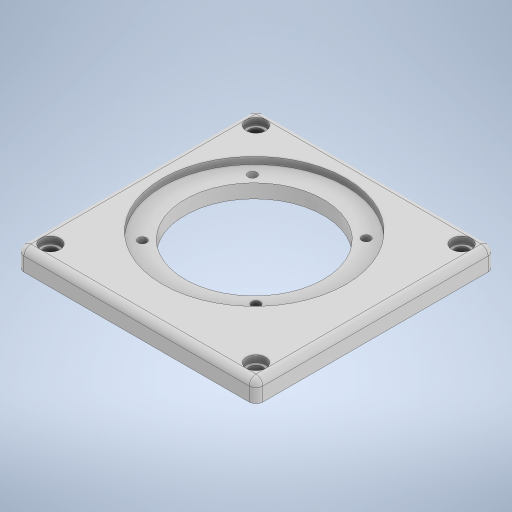
# Autodesk Inventor part: joystickBOXtop
Saved by Autodesk Inventor 2023 (Build 270158000, 158)
## iProperties
Created: 2023-09-26
Part Number: joystickBOXtop
Material: Generic
Document SubType Name: Modeling
Designer: Nikita
Density: 1 g/cm^3
Appearance: Default
Author: Nikita
Autodesk Inventor part; units mm, degrees
ref_plane "YZ Plane" through (0, 0, 0) normal (1, 0, 0) x (0, 1, 0)
ref_plane "XZ Plane" through (0, 0, 0) normal (0, 1, 0) x (-1, 0, 0)
ref_plane "XY Plane" through (0, 0, 0) normal (0, 0, 1) x (1, 0, 0)
sketch "Sketch1" plane through (0, 0, 0) normal (0, 1, 0) x (-1, 0, 0)
  line L0 (0, 0) -> (69, 0)
  line L1 (69, 0) -> (69, -69)
  line L2 (69, -69) -> (0, -69)
  line L3 (0, -69) -> (0, 0)
  dimension "d0" = 69
  dimension "d1" = 69
  constraints: 8 end point, 3 perpendicular, 1 horizontal
  measures "d0" distance of L0.start L0.end
  measures "d1" distance of L0.end L1.end
extrude "Extrusion1" add sketch "Sketch1" along normal blind 6
sketch "Sketch2" plane through (0, 6, 0) normal (0, 1, 0) x (1, 0, 0)
  line L0 (0, 0) -> (0, 69) construction
  line L1 (0, 69) -> (-69, 69) construction
  line L2 (0, 0) -> (-69, 69) construction
  line L3 (-69, 69) -> (-69, 0) construction
  line L4 (-69.6585, 0.6585) -> (-0.6585, 69.6585) construction
  circle A0 centre (-37.9036, 37.4036) radius 20
  line L5 (-61.9507, 69) -> (-61.9507, 54) construction
  line L6 (-37.9036, 17.4036) -> (-58.9036, 17.4036) construction
  line L7 (-58.9036, 17.4036) -> (-17.4036, 17.4036) construction
  line L8 (-58.4036, 17.4036) -> (-58.4036, 58.5866) construction
  line L9 (-58.4036, 58.5866) -> (-17.4036, 58.5866) construction
  line L10 (-17.4036, 58.5866) -> (-17.4036, 17.4036) construction
  line L11 (-69, 69) -> (-69, 0) construction
  line L12 (-69, 54) -> (-54, 54) construction
  line L13 (-69, 69) -> (-37.9036, 37.9036)
  dimension "d4" = 40
  dimension "d55" = 15
  dimension "d65" = 43.977
  constraints: 22 end point, 4 horizontal, 4 point on line, 2 perpendicular, 1 parallel, 1 vertical, 1 vertical alignment, 2 other
  measures "d55" distance of L5.start L5.end
  measures "d65" distance of L1.end L13.end
extrude "Extrusion2" cut sketch "Sketch2" against normal blind 6
fillet "Fillet1" radius 2 1 edges at (-34.5, 6, 0)
fillet "Fillet2" radius 2 3 edges at (0, 6, -35.5) (0, 5.4142, -0.5858) (0, 2, 0)
fillet "Fillet3" radius 2 3 edges at (-0.5858, 5.4142, -69) (0, 2, -69) (-35.5, 6, -69)
fillet "Fillet4" radius 2 5 edges at (-69, 5.4142, -0.5858) (-69, 2, 0) (-69, 5.4142, -68.4142) (-69, 2, -69) (-69, 6, -34.5)
sketch "Sketch3" plane through (0, 6, 0) normal (0, 1, 0) x (1, 0, 0)
  line L0 (-67, 69) -> (-67, 67) construction
  line L1 (-2, 2) -> (-67, 2) construction
  line L2 (-67, 67) -> (-2, 67) construction
  line L3 (-67, 2) -> (-67, 67) construction
  circle A0 centre (-22, 53.808) radius 1.25
  line L4 (-69, 67) -> (-69, 2) construction
  circle A1 centre (-37.9036, 37.4036) radius 20 construction
  line L5 (-17.9036, 37.4036) -> (-17.9036, 58.4036) construction
  line L6 (-22, 53.808) -> (-54, 53.808) construction
  line L7 (-22, 21.808) -> (-54, 21.808) construction
  line L8 (-54, 21.808) -> (-54, 53.808) construction
  line L9 (-22, 53.808) -> (-22, 21.808) construction
  line L10 (-22, 53.808) -> (-54, 21.808) construction
  line L11 (-69, 59.0495) -> (-54, 59.0495) construction
  line L12 (-54, 69) -> (-54, 53.808) construction
  point P0 (0, 0)
  dimension "d14" = 2.5
  dimension "d63" = 32
  dimension "d64" = 15
  constraints: 16 end point, 2 horizontal, 1 centre point, 1 horizontal alignment, 1 parallel, 1 perpendicular, 1 point on line, 1 vertical, 1 other
  measures "d14" diameter of A0
  measures "d63" distance of L6.start L6.end
  measures "d64" distance of L11.start L11.end
extrude "Extrusion3" cut sketch "Sketch3" against normal blind 10
pattern_circular "Circular Pattern1" count 4 over 360 about axis through (-37.9036, 6, -37.4036) along (0, -1, 0) of "Extrusion3"
sketch "Sketch6" plane through (0, 6, 0) normal (0, 1, 0) x (1, 0, 0)
  line L0 (-2, 67) -> (-2, 2) projected
  arc A0 (-2, 0) -> (0, 2) centre (-2, 2) ccw projected
  line L1 (0, 2) -> (-2, 2) projected
  line L2 (0, 0) -> (-2, 2)
  line L3 (-0.5858, 0.5858) -> (-4.8284, 4.8284) construction
  circle A1 centre (-4.8284, 4.8284) radius 2
  dimension "d52" = 6
  dimension "d53" = 4
  constraints: 4 end point, 2 point on line, 1 centre point, 1 coincident, 1 point on circle
  measures "d52" distance of L3.start L3.end
  measures "d53" diameter of A1
extrude "Extrusion5" cut sketch "Sketch6" against normal blind 18.75 contours A1
pattern_linear "Rectangular Pattern1" count 2 spacing 59.343 along (0, 0, -1) count 2 spacing 59.343 along (-1, 0, 0) of "Extrusion5"
sketch "Sketch8" plane through (0, 6, 0) normal (0, 1, 0) x (1, 0, 0)
  line L0 (-2, 2) -> (-67, 2) projected
  circle A0 centre (-4.8284, 4.8284) radius 2 construction
  line L1 (-4.8284, 4.8284) -> (-2, 2) construction
  circle A1 centre (-4.8284, 4.8284) radius 2.8284 construction
  circle A2 centre (-4.8284, 4.8284) radius 2.8284
  circle A3 centre (-4.8284, 4.8284) radius 2
  point P0 (0, 0)
  point P1 (-4.1213, 4.1213)
  constraints: 3 centre point, 3 coincident, 2 concentric, 2 end point, 1 tangent
extrude "Extrusion6" cut sketch "Sketch8" against normal blind 2 contours A2 | A3
pattern_linear "Rectangular Pattern2" count 2 spacing 59.343 along (-1, 0, 0) count 2 spacing 59.343 along (0, 0, -1) of "Extrusion6"
sketch "Sketch9" plane through (0, 6, 0) normal (0, 1, 0) x (1, 0, 0)
  circle A0 centre (-37.9036, 37.4036) radius 20 projected
  circle A1 centre (-37.9036, 37.4036) radius 26.5
  point P0 (0, 0)
  dimension "d59" = 53
  constraints: 1 centre point, 1 coincident
  measures "d59" diameter of A1
extrude "Extrusion7" cut sketch "Sketch9" against normal blind 2
equation "\"d0\" = d1"
body "Solid1"
